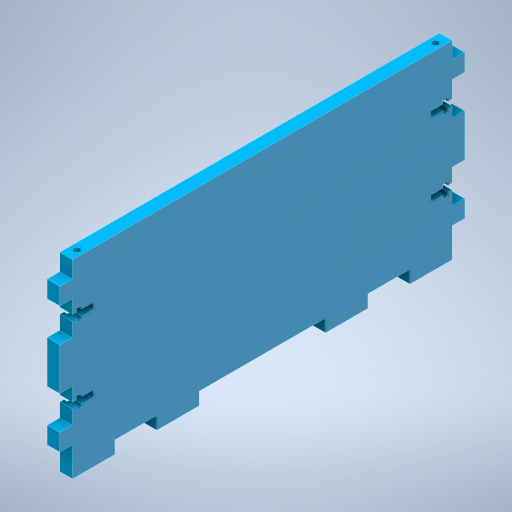
# Autodesk Inventor part: передняя стенка
Saved by Autodesk Inventor 2024.2 (Build 282272000, 272)
## iProperties
Created: 2025-11-20
Part Number: передняя стенка
Material: Типовые
Document SubType Name: Modeling
Designer: Zakhar
Density: 1 g/cm^3
Appearance: Небесно-голубой — нейтральный
Mass: 95.616 g
Surface Area: 351.84 cm^2
Volume: 95.616 cm^3
Author: Zakhar
Autodesk Inventor part; units mm, degrees
ref_plane "YZ Plane" through (0, 0, 0) normal (1, 0, 0) x (0, 1, 0)
ref_plane "XZ Plane" through (0, 0, 0) normal (0, 1, 0) x (-1, 0, 0)
ref_plane "XY Plane" through (0, 0, 0) normal (0, 0, 1) x (1, 0, 0)
sketch "Эскиз1" plane through (0, 0, 0) normal (1, 0, 0) x (0, 1, 0)
  line L0 (84, 90) -> (0, 90)
  line L1 (0, 90) -> (0, -90)
  line L2 (0, -90) -> (84, -90)
  line L3 (84, -90) -> (84, 90)
  line L4 (76, 90) -> (8, 90)
  line L5 (8, 90) -> (8, 96)
  line L6 (8, 96) -> (76, 96)
  line L7 (76, 96) -> (76, 90)
  line L8 (76, -90) -> (8, -90)
  line L9 (8, -90) -> (8, -96)
  line L10 (8, -96) -> (76, -96)
  line L11 (76, -96) -> (76, -90)
  line L12 (16, -96) -> (16, -90)
  line L13 (32, -96) -> (32, -90)
  line L14 (68, -96) -> (68, -90)
  line L15 (52, -96) -> (52, -90)
  line L16 (16, 90) -> (16, 96)
  line L17 (32, 90) -> (32, 96)
  line L18 (68, 90) -> (68, 96)
  line L19 (52, 90) -> (52, 96)
  circle A0 centre (20, -59.5) radius 1.5
  circle A1 centre (20, -73.5) radius 1.5
  circle A2 centre (7, -59.5) radius 1.5
  circle A3 centre (7, -73.5) radius 1.5
  line L20 (20, -59.5) -> (0, -59.5) construction
  line L21 (7, -59.5) -> (7, -73.5) construction
  line L22 (20, -73.5) -> (0, -73.5) construction
  point P0 (0, 0)
  point P1 (76, 93)
  point P2 (8, 93)
  point P3 (8, -90)
  point P4 (68, -93)
  point P5 (76, -93)
  point P6 (52, -93)
  point P7 (16, -93)
  point P8 (8, -93)
  point P9 (32, -93)
  point P10 (68, 93)
  point P11 (52, 93)
  point P12 (16, 93)
  point P13 (32, 93)
  dimension "d0" = 180
  dimension "d1" = 84
  dimension "d2" = 90
  dimension "d3" = 0
  dimension "d4" = 6
  dimension "d5" = 8
  dimension "d6" = 8
  dimension "d7" = 6
  dimension "d40" = 8
  dimension "d41" = 16
  dimension "d42" = 8
  dimension "d43" = 16
  dimension "d44" = 8
  dimension "d45" = 16
  dimension "d46" = 16
  dimension "d47" = 8
  dimension "d76" = 14
  dimension "d77" = 3
  dimension "d78" = 3
  dimension "d79" = 20
  dimension "d80" = 20
  dimension "d81" = 3
  dimension "d82" = 3
  dimension "d83" = 13
  dimension "d84" = 13
  dimension "d85" = 16.5
  constraints: 46 end point, 24 point on line, 13 perpendicular, 12 midpoint, 6 parallel, 4 centre point, 3 horizontal
  measures "d0" distance of L0.end L1.end
  measures "d1" distance of L0.start L0.end
  measures "d2" distance from line of point (0, 0) L2
  measures "d3" distance from line of L1 point (0, 0)
  measures "d4" distance of L6.end L4.start
  measures "d5" horizontal distance of L0.start point (76, 93)
  measures "d6" horizontal distance of L0.end point (8, 93)
  measures "d7" distance between parallel lines of L2 L10
  measures "d40" distance of point (68, -93) point (76, -93)
  measures "d41" distance of point (52, -93) point (68, -93)
  measures "d42" distance of point (16, -93) point (8, -93)
  measures "d43" distance of point (32, -93) point (16, -93)
  measures "d44" distance of point (76, 93) point (68, 93)
  measures "d45" distance of point (52, 93) point (68, 93)
  measures "d46" distance of point (16, 93) point (32, 93)
  measures "d47" distance of point (8, 93) point (16, 93)
  measures "d76" distance of L22.start L20.start
  measures "d77" diameter of A0
  measures "d78" diameter of A1
  measures "d79" distance from line of L1 L20.start
  measures "d80" distance from line of L1 L22.start
  measures "d81" diameter of A3
  measures "d82" diameter of A2
  measures "d83" distance of L20.start L21.start
  measures "d84" distance of L22.start L21.end
  measures "d85" distance from line of L8 L22.start
extrude "Выдавливание1" add sketch "Эскиз1" along normal blind 6 contours L3 L2 L1 L0 | L0 L18 L6 L7 | L11 L10 L14 L2 | L0 L17 L6 L19 | L15 L10 L13 L2 | L0 L5 L6 L16 | L12 L10 L9 L2 | A0 | A1 | A2 | A3
sketch "Эскиз4" plane through (0, 84, 90) normal (0, 1, 0) x (1, 0, 0)
  circle A0 centre (3, 5) radius 1.5
  circle A1 centre (3, 175) radius 1.5
  line L0 (0, 0) -> (6, 0)
  line L1 (6, 180) -> (6, 0)
  line L2 (0, 180) -> (6, 180)
  line L3 (6, 180) -> (6, 0) projected
  line L4 (0, 0) -> (6, 0) projected
  line L5 (0, 180) -> (6, 180) projected
  point P0 (0, 90)
  point P1 (3, 0)
  dimension "d30" = 3
  dimension "d31" = 3
  dimension "d32" = 5
  dimension "d33" = 3
  dimension "d34" = 5
  dimension "d35" = 3
  dimension "d36" = 6
  dimension "d37" = 6
  constraints: 6 end point, 3 collinear, 2 centre point, 1 midpoint
  measures "d30" diameter of A1
  measures "d31" diameter of A0
  measures "d32" distance of point (3, 0) A0.centre
  measures "d33" distance from line of L1 A0.centre
  measures "d34" distance from line of L2 A1.centre
  measures "d35" distance from line of L1 A1.centre
  measures "d36" distance of L2.start L1.start
  measures "d37" distance of L0.start L0.end
extrude "Выдавливание4" cut sketch "Эскиз4" against normal blind 4
sketch "Эскиз6" plane through (6, 0, 0) normal (1, 0, 0) x (0, 0, -1)
  line L0 (-90, 8) -> (-90, 0) projected
  line L1 (-90, 0) -> (-70, 0)
  line L2 (-70, 0) -> (-70, -6)
  line L3 (-70, -6) -> (-90, -6)
  line L4 (-90, -6) -> (-90, 0)
  line L5 (-90, 0) -> (90, 0) projected
  line L6 (-50, 0) -> (-30, 0)
  line L7 (-30, 0) -> (-30, -6)
  line L8 (-30, -6) -> (-50, -6)
  line L9 (-50, -6) -> (-50, 0)
  line L10 (30, 0) -> (50, 0)
  line L11 (50, 0) -> (50, -6)
  line L12 (50, -6) -> (30, -6)
  line L13 (30, -6) -> (30, 0)
  line L14 (90, 0) -> (70, 0)
  line L15 (70, 0) -> (70, -6)
  line L16 (70, -6) -> (90, -6)
  line L17 (90, -6) -> (90, 0)
  point P0 (0, 0)
  point P1 (-80, -6)
  point P2 (-50, -3)
  point P3 (-70, -3)
  point P4 (-30, -3)
  point P5 (90, -3)
  point P6 (70, -3)
  point P7 (50, -3)
  dimension "d48" = 6
  dimension "d49" = 6
  dimension "d50" = 6
  dimension "d51" = 20
  dimension "d52" = 20
  dimension "d53" = 20
  dimension "d54" = 20
  dimension "d55" = 20
  dimension "d56" = 20
  constraints: 32 end point, 8 parallel, 7 midpoint, 4 horizontal, 4 perpendicular, 3 point on line
  measures "d48" distance from line of L5 point (-80, -6)
  measures "d49" distance of L6.end L7.end
  measures "d50" distance of L12.end L10.start
  measures "d51" distance of L2.end L3.end
  measures "d52" distance of point (-50, -3) point (-70, -3)
  measures "d53" distance of point (-30, -3) point (-50, -3)
  measures "d54" distance of point (90, -3) point (70, -3)
  measures "d55" distance of point (70, -3) point (50, -3)
  measures "d56" distance from line of point (50, -3) L13
extrude "Выдавливание5" add sketch "Эскиз6" against normal blind 6
sketch "Эскиз8" plane through (6, 0, 0) normal (1, 0, 0) x (0, 0, -1)
  line L0 (90, 60) -> (80, 60)
  line L1 (80, 60) -> (80, 57)
  line L2 (80, 57) -> (90, 57)
  line L3 (90, 57) -> (90, 60)
  line L4 (85.6, 55.5) -> (88, 55.5)
  line L5 (88, 55.5) -> (88, 61.5)
  line L6 (88, 61.5) -> (85.6, 61.5)
  line L7 (85.6, 61.5) -> (85.6, 55.5)
  line L8 (90, 25.5) -> (80, 25.5)
  line L9 (80, 25.5) -> (80, 22.5)
  line L10 (80, 22.5) -> (90, 22.5)
  line L11 (90, 22.5) -> (90, 25.5)
  line L12 (85.6, 27) -> (88, 27)
  line L13 (88, 27) -> (88, 21)
  line L14 (88, 21) -> (85.6, 21)
  line L15 (85.6, 21) -> (85.6, 27)
  line L16 (-85.6, 27) -> (-88, 27)
  line L17 (-90, 22.5) -> (-90, 25.5)
  line L18 (-85.6, 21) -> (-85.6, 27)
  line L19 (-88, 21) -> (-85.6, 21)
  line L20 (-88, 27) -> (-88, 21)
  line L21 (-80, 61.5) -> (-80, 58.5)
  line L22 (-90, 61.5) -> (-80, 61.5)
  line L23 (-80, 25.5) -> (-80, 22.5)
  line L24 (-90, 25.5) -> (-80, 25.5)
  line L25 (-80, 22.5) -> (-90, 22.5)
  line L26 (-80, 58.5) -> (-90, 58.5)
  line L27 (-85.6, 57) -> (-88, 57)
  line L28 (-90, 58.5) -> (-90, 61.5)
  line L29 (-88, 57) -> (-88, 63)
  line L30 (-85.6, 63) -> (-85.6, 57)
  line L31 (-88, 63) -> (-85.6, 63)
  line L32 (90, 32) -> (96, 32) projected
  line L33 (90, 16) -> (90, 32) projected
  line L34 (90, 68) -> (96, 68) projected
  line L35 (-96, 68) -> (-90, 68) projected
  line L36 (-90, 68) -> (-90, 52) projected
  line L37 (-90, 32) -> (-90, 16) projected
  line L38 (-96, 32) -> (-90, 32) projected
  point P0 (0, 0)
  point P1 (97.0761, 73.2611)
  point P2 (97.0761, 37.2611)
  point P3 (-93, 32)
  point P4 (85.6, 22.5)
  point P5 (88, 22.5)
  point P6 (88, 25.5)
  point P7 (85.6, 25.5)
  point P8 (85.6, 57)
  point P9 (88, 57)
  point P10 (88, 60)
  point P11 (85.6, 60)
  point P12 (-88, 25.5)
  point P13 (-88, 22.5)
  point P14 (-85.6, 22.5)
  point P15 (-85.6, 25.5)
  point P16 (-85.6, 61.5)
  point P17 (-88, 61.5)
  point P18 (-88, 58.5)
  point P19 (-85.6, 58.5)
  dimension "d86" = 6
  dimension "d87" = 2.4
  dimension "d88" = 10
  dimension "d89" = 3
  dimension "d90" = 1.5
  dimension "d91" = 5.6
  dimension "d92" = 10
  dimension "d93" = 3
  dimension "d94" = 1.5
  dimension "d95" = 6
  dimension "d96" = 5.6
  dimension "d97" = 2.4
  dimension "d100" = 6.5
  dimension "d101" = 10
  dimension "d102" = 8
  dimension "d103" = 6.5
  dimension "d104" = 3
  dimension "d105" = 10
  dimension "d106" = 2.4
  dimension "d107" = 1.5
  dimension "d108" = 6
  dimension "d109" = 2
  dimension "d110" = 6
  dimension "d111" = 2.4
  dimension "d112" = 10
  dimension "d113" = 3
  dimension "d114" = 6.5
  dimension "d115" = 1.5
  constraints: 64 end point, 15 perpendicular, 8 parallel, 4 horizontal, 2 collinear, 2 point on line, 1 midpoint
  measures "d86" distance between parallel lines of L14 L12
  measures "d87" distance between parallel lines of L15 L13
  measures "d88" distance of L9.end L11.start
  measures "d89" distance between parallel lines of L8 L10
  measures "d90" distance between parallel lines of L10 L14
  measures "d91" distance between parallel lines of L9 L15
  measures "d92" distance of L1.end L3.start
  measures "d93" distance of L3.start L3.end
  measures "d94" distance between parallel lines of L0 L6
  measures "d95" distance of L4.end L5.end
  measures "d96" distance between parallel lines of L1 L7
  measures "d97" distance of L4.start L4.end
  measures "d100" distance between parallel lines of L8 L32
  measures "d101" distance between parallel lines of L33 L9
  measures "d102" distance between parallel lines of L34 L0
  measures "d103" distance between parallel lines of L35 L22
  measures "d104" distance of L22.end L26.start
  measures "d105" distance of L26.start L28.start
  measures "d106" distance of L31.start L31.end
  measures "d107" distance between parallel lines of L22 L31
  measures "d108" distance of L29.start L31.start
  measures "d109" distance between parallel lines of L28 L29
  measures "d110" distance of L19.end L16.start
  measures "d111" distance of L16.start L16.end
  measures "d112" distance of L17.end L24.end
  measures "d113" distance of L24.end L25.start
  measures "d114" distance from line of L24 point (-93, 32)
  measures "d115" distance between parallel lines of L25 L19
extrude "Выдавливание7" cut sketch "Эскиз8" against normal blind 10
equation "\"d2\" = 0.5 * d0"
equation "\"d42\" = d40"
equation "\"d43\" = d41"
equation "\"d44\" = d40"
equation "\"d45\" = d41"
equation "\"d46\" = d41"
equation "\"d47\" = d40"
equation "\"d52\" = d51"
equation "\"d53\" = d51"
equation "\"d54\" = d51"
equation "\"d55\" = d51"
equation "\"d56\" = d51"
